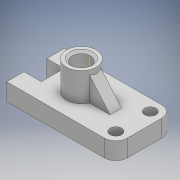
# Autodesk Inventor part: Основание
Saved by Autodesk Inventor 2018 (Build 220112000, 112)
## iProperties
Created: 2018-05-16
Part Number: Основание
Material: Типовые
Document SubType Name: Modeling
Designer: user
Density: 1 g/cm^3
Appearance: По умолчанию
Author: user
Autodesk Inventor part; units mm, degrees
ref_plane "YZ Plane" through (0, 0, 0) normal (1, 0, 0) x (0, 1, 0)
ref_plane "XZ Plane" through (0, 0, 0) normal (0, 1, 0) x (-1, 0, 0)
ref_plane "XY Plane" through (0, 0, 0) normal (0, 0, 1) x (1, 0, 0)
sketch "Эскиз1" plane through (0, 0, 0) normal (0, 0, 1) x (1, 0, 0)
  line L0 (-47.5, -25) -> (47.5, -25)
  line L1 (47.5, -25) -> (47.5, 25)
  line L2 (47.5, 25) -> (-47.5, 25)
  line L3 (-47.5, 25) -> (-47.5, -25)
  line L4 (-47.5, -25) -> (47.5, 25) construction
  line L5 (47.5, -25) -> (-47.5, 25) construction
  point P0 (0, 0)
  dimension "d0" = 95
  dimension "d1" = 50
  constraints: 12 end point, 2 midpoint, 2 parallel, 1 horizontal, 1 perpendicular
  measures "d0" distance of L2.end L1.end
  measures "d1" distance of L1.end L0.end
extrude "Выдавливание1" add sketch "Эскиз1" along normal blind 15
sketch "Эскиз2" plane through (-47.5, -25, 0) normal (-1, 0, 0) x (0, 0, 1)
  point P0 (0, 25)
sketch "Эскиз3" plane through (-47.5, -25, 0) normal (-1, 0, 0) x (0, 0, 1)
  line L0 (15, 0) -> (15, 50) projected
  line L1 (0, 35) -> (15, 35)
  line L2 (15, 35) -> (15, 15)
  line L3 (15, 15) -> (0, 15)
  line L4 (0, 15) -> (0, 35)
  line L5 (0, 25) -> (15, 25)
  dimension "d4" = 20
  constraints: 10 end point, 2 horizontal, 2 parallel, 1 midpoint, 1 perpendicular, 1 point on line, 1 other
  measures "d4" distance of L3.end L1.start
extrude "Выдавливание2" cut sketch "Эскиз3" against normal blind 15
fillet "Сопряжение1" radius 10 1 edges at (47.5, 25, 7.5)
fillet "Сопряжение2" radius 10 1 edges at (47.5, -25, 7.5)
sketch "Эскиз4" plane through (0, 0, 15) normal (0, 0, 1) x (1, 0, 0)
  line L0 (0, 0) -> (47.5, 0)
  line L1 (47.5, -15) -> (47.5, 15) projected
  line L2 (-47.5, 25) -> (-47.5, 10) projected
  point P0 (37.5, 15)
  point P1 (37.5, -15)
  dimension "d9" = 30
  dimension "d10" = 85
  constraints: 2 end point, 1 midpoint, 1 symmetric about line
  measures "d9" distance of point (37.5, -15) point (37.5, 15)
  measures "d10" distance from line of L2 point (37.5, 15)
hole "Отверстие1" at (37.5, 15, 15) at (37.5, -15, 15) direction (0, 0, -1) diameter 10 end through all
sketch "Эскиз5" plane through (0, 0, 15) normal (0, 0, 1) x (1, 0, 0)
  circle A0 centre (-7.5, 0) radius 13
  line L0 (-47.5, 25) -> (-47.5, 10) projected
  point P0 (0, 0)
  dimension "d18" = 26
  dimension "d19" = 40
  constraints: 1 centre point
  measures "d18" diameter of A0
  measures "d19" distance from line of L0 A0.centre
extrude "Выдавливание3" add sketch "Эскиз5" along normal blind 25
sketch "Эскиз6" plane through (-7.5, 0, 40) normal (0, 0, 1) x (1, 0, 0)
  point P0 (7.5, 0)
  point P1 (0, 0)
hole "Отверстие2" at (-7.5, 0, 40) direction (0, 0, -1) diameter 16 depth 30 tip angle 118 clearance for "болты с шестигранной головкой / гайка ГОСТ 12876-67" size "M16" standard "ГОСТ"
chamfer "Фаска1" distance 2 angle 45 1 edges at (-7.5, 8, 40)
sketch "Эскиз7" plane through (0, 0, 15) normal (0, 0, 1) x (1, 0, 0)
  point P0 (0, 0)
sketch "Эскиз8" plane through (0, 0, 0) normal (0, 1, 0) x (-1, 0, 0)
  line L0 (20.5, 40) -> (-5.5, 40) projected
  line L1 (0, 40) -> (-11.4909, 40)
  line L2 (-11.4909, 40) -> (-5.5, 35)
  line L3 (-5.5, 15) -> (-5.5, 40) projected
  line L4 (-5.5, 35) -> (-22.5, 15)
  line L5 (47.5, 0) -> (47.5, 15) projected
  line L6 (-22.5, 15) -> (47.5, 15)
  line L7 (-5.5, 35) -> (-1.25, 40)
  line L8 (17.5, 40) -> (-2.5, 40) projected
  line L9 (-2.5, 40) -> (-0.5, 38) projected
  line L10 (-1.8243, 39.3243) -> (-1.8243, 15)
  line L11 (-37.5, 15) -> (47.5, 15) projected
  point P0 (0, 0)
  dimension "d32" = 70
  dimension "d33" = 5
  constraints: 12 end point, 6 point on line, 2 perpendicular, 1 collinear
  measures "d32" distance of L4.end L5.end
  measures "d33" distance from line of L1 L2.end
extrude "Выдавливание4" add sketch "Эскиз8" along normal mid plane 10 contours L10 L6 L3 L7 | L3 L6 L4
